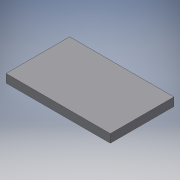
# Autodesk Inventor part: Base supp.saldato
Saved by Autodesk Inventor 2018 (Build 220112000, 112)
## iProperties
Created: 2020-06-01
Part Number: Base supp.saldato
Material: Generico
Document SubType Name: Modeling
Designer: Francesco
Density: 1 g/cm^3
Appearance: Default
Author: Francesco
Autodesk Inventor part; units mm, degrees
ref_plane "YZ Plane" through (0, 0, 0) normal (1, 0, 0) x (0, 1, 0)
ref_plane "XZ Plane" through (0, 0, 0) normal (0, 1, 0) x (-1, 0, 0)
ref_plane "XY Plane" through (0, 0, 0) normal (0, 0, 1) x (1, 0, 0)
sketch "Schizzo1" plane through (0, 0, 0) normal (0, 0, 1) x (1, 0, 0)
  line L0 (-50, 30.5) -> (50, 30.5)
  line L1 (50, 30.5) -> (50, -30.5)
  line L2 (50, -30.5) -> (-50, -30.5)
  line L3 (-50, -30.5) -> (-50, 30.5)
  line L4 (-50, 30.5) -> (50, -30.5) construction
  line L5 (50, 30.5) -> (-50, -30.5) construction
  point P0 (0, 0)
  dimension "d0" = 100
  dimension "d1" = 61
  constraints: 12 end point, 2 midpoint, 2 parallel, 1 horizontal, 1 perpendicular
  measures "d0" distance of L1.end L2.end
  measures "d1" distance of L0.end L1.end
extrude "Estrusione1" add sketch "Schizzo1" along normal blind 8
